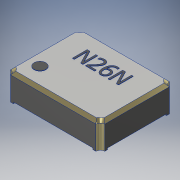
# Autodesk Inventor part: Crystal_TXO-3225
Saved by Autodesk Inventor 2018 (Build 220112000, 112)
## iProperties
Created: 2016-08-15
Part Number: Crystal_TXO-3225
Material: Aluminum 6061
Document SubType Name: Modeling
Designer: Bradley
Density: 2.7 g/cm^3
Appearance: Aluminum - Flat
Author: Bradley
Autodesk Inventor part; units mm, degrees
ref_plane "YZ Plane" through (0, 0, 0) normal (1, 0, 0) x (0, 1, 0)
ref_plane "XZ Plane" through (0, 0, 0) normal (0, 1, 0) x (-1, 0, 0)
ref_plane "XY Plane" through (0, 0, 0) normal (0, 0, 1) x (1, 0, 0)
sketch "Sketch1" plane through (0, 0, 0) normal (0, 1, 0) x (-1, 0, 0)
  line L0 (-1.6, 1.25) -> (1.6, 1.25)
  line L1 (1.6, 1.25) -> (1.6, -1.25)
  line L2 (1.6, -1.25) -> (-1.6, -1.25)
  line L3 (-1.6, -1.25) -> (-1.6, 1.25)
  line L4 (-1.6, 1.25) -> (1.6, -1.25) construction
  line L5 (1.6, 1.25) -> (-1.6, -1.25) construction
  arc A0 (1.6, -1.1) -> (1.45, -1.25) centre (1.6, -1.25) ccw
  arc A1 (-1.45, -1.25) -> (-1.6, -1.1) centre (-1.6, -1.25) ccw
  arc A2 (-1.6, 1.1) -> (-1.45, 1.25) centre (-1.6, 1.25) ccw
  arc A3 (1.45, 1.25) -> (1.6, 1.1) centre (1.6, 1.25) ccw
  point P0 (0, 0)
  dimension "d0" = 3.2
  dimension "d1" = 2.5
  dimension "d4" = 0.15
  constraints: 12 end point, 8 point on circle, 8 point on line, 4 centre point, 4 coincident, 3 equal radius, 2 midpoint, 2 parallel, 1 horizontal, 1 perpendicular
  measures "d0" distance of L1.end L2.end
  measures "d1" distance of L0.end L1.end
  measures "d4" radius of A0
extrude "Extrusion1" add sketch "Sketch1" along normal mid plane 0.85 contours L0 A3 L1 A0 L2 A1 L3 A2
chamfer "Chamfer1" distance 0.1 angle 45 8 edges at (0, 0.425, 1.25) (-1.4939, 0.425, 1.1439) (-1.6, 0.425, 0) (-1.4939, 0.425, -1.1439) (0, 0.425, -1.25) (1.4939, 0.425, -1.1439) (1.6, 0.425, 0) (1.4939, 0.425, 1.1439)
sketch "Sketch3" plane through (0, 0.425, 0) normal (0, 1, 0) x (1, 0, 0)
  line L0 (-1.3709, 1.15) -> (1.3709, 1.15) projected
  arc A0 (-1.5, 1.0209) -> (-1.3709, 1.15) centre (-1.6, 1.25) ccw projected
  line L1 (-1.5, -1.0209) -> (-1.5, 1.0209) projected
  arc A1 (-1.3709, -1.15) -> (-1.5, -1.0209) centre (-1.6, -1.25) ccw projected
  line L2 (1.3709, -1.15) -> (-1.3709, -1.15) projected
  arc A2 (1.5, -1.0209) -> (1.3709, -1.15) centre (1.6, -1.25) ccw projected
  line L3 (1.5, 1.0209) -> (1.5, -1.0209) projected
  arc A3 (1.3709, 1.15) -> (1.5, 1.0209) centre (1.6, 1.25) ccw projected
  line L4 (1.5, 1.0209) -> (1.5, -1.0209) construction
  line L5 (1.5, 0.1868) -> (-1.5, 0.1868) construction
  circle A4 centre (-1.1, -0.6) radius 0.2
  line L6 (-0.4259, 0.1868) -> (-0.5004, 0.1868)
  line L7 (-0.5004, 0.1868) -> (-0.7216, 0.6179)
  line L8 (-0.7216, 0.6179) -> (-0.7216, 0.1868)
  line L9 (-0.7216, 0.1868) -> (-0.7836, 0.1868)
  line L10 (-0.7836, 0.1868) -> (-0.7836, 0.6868)
  line L11 (-0.7836, 0.6868) -> (-0.6892, 0.6868)
  line L12 (-0.6892, 0.6868) -> (-0.4878, 0.2909)
  line L13 (-0.4878, 0.2909) -> (-0.4878, 0.6868)
  line L14 (-0.4878, 0.6868) -> (-0.4259, 0.6868)
  line L15 (-0.4259, 0.6868) -> (-0.4259, 0.1868)
  line L16 (-0.0304, 0.1868) -> (-0.3387, 0.1868)
  line L17 (-0.3387, 0.1868) -> (-0.3387, 0.2577)
  spline S0 degree 2 poles (-0.3387, 0.2577) (-0.3055, 0.2889) (-0.2464, 0.3468) (-0.218, 0.378) knots 0 0 0 1 2 2 2
  spline S1 degree 2 poles (-0.218, 0.378) (-0.1609, 0.4408) (-0.1191, 0.5162) (-0.1191, 0.5563) knots 0 0 0 1 2 2 2
  spline S2 degree 2 poles (-0.1191, 0.5563) (-0.1191, 0.5774) (-0.1321, 0.609) (-0.1438, 0.6191) knots 0 0 0 1 2 2 2
  spline S3 degree 2 poles (-0.1438, 0.6191) (-0.1556, 0.6292) (-0.1864, 0.6393) (-0.205, 0.6393) knots 0 0 0 1 2 2 2
  spline S4 degree 2 poles (-0.205, 0.6393) (-0.2229, 0.6393) (-0.2593, 0.6304) (-0.2759, 0.6235) knots 0 0 0 1 2 2 2
  spline S5 degree 2 poles (-0.2759, 0.6235) (-0.2901, 0.6179) (-0.3165, 0.6017) (-0.3246, 0.596) knots 0 0 0 1 2 2 2
  line L18 (-0.3246, 0.596) -> (-0.3282, 0.596)
  line L19 (-0.3282, 0.596) -> (-0.3282, 0.6673)
  spline S6 degree 2 poles (-0.3282, 0.6673) (-0.3075, 0.6774) (-0.2334, 0.6973) (-0.2002, 0.6973) knots 0 0 0 1 2 2 2
  spline S7 degree 2 poles (-0.2002, 0.6973) (-0.1301, 0.6973) (-0.0511, 0.6231) (-0.0511, 0.5599) knots 0 0 0 1 2 2 2
  spline S8 degree 2 poles (-0.0511, 0.5599) (-0.0511, 0.5304) (-0.0648, 0.4809) (-0.077, 0.4599) knots 0 0 0 1 2 2 2
  spline S9 degree 2 poles (-0.077, 0.4599) (-0.0891, 0.438) (-0.1244, 0.395) (-0.1438, 0.3744) knots 0 0 0 1 2 2 2
  spline S10 degree 2 poles (-0.1438, 0.3744) (-0.1754, 0.3399) (-0.2528, 0.2662) (-0.2759, 0.2447) knots 0 0 0 1 2 2 2
  line L20 (-0.2759, 0.2447) -> (-0.0304, 0.2447)
  line L21 (-0.0304, 0.2447) -> (-0.0304, 0.1868)
  spline S11 degree 2 poles (0.3525, 0.3488) (0.3525, 0.3103) (0.327, 0.2451) (0.3055, 0.2232) knots 0 0 0 1 2 2 2
  spline S12 degree 2 poles (0.3055, 0.2232) (0.2832, 0.2001) (0.2273, 0.1762) (0.1937, 0.1762) knots 0 0 0 1 2 2 2
  spline S13 degree 2 poles (0.1937, 0.1762) (0.16, 0.1762) (0.1045, 0.1989) (0.0835, 0.2216) knots 0 0 0 1 2 2 2
  spline S14 degree 2 poles (0.0835, 0.2216) (0.0575, 0.2488) (0.0284, 0.3399) (0.0284, 0.4064) knots 0 0 0 1 2 2 2
  spline S15 degree 2 poles (0.0284, 0.4064) (0.0284, 0.4716) (0.0551, 0.5765) (0.0831, 0.6154) knots 0 0 0 1 2 2 2
  spline S16 degree 2 poles (0.0831, 0.6154) (0.1102, 0.6535) (0.1961, 0.6961) (0.2524, 0.6961) knots 0 0 0 1 2 2 2
  spline S17 degree 2 poles (0.2524, 0.6961) (0.269, 0.6961) (0.2982, 0.6928) (0.3092, 0.6892) knots 0 0 0 1 2 2 2
  line L22 (0.3092, 0.6892) -> (0.3092, 0.6248)
  line L23 (0.3092, 0.6248) -> (0.3063, 0.6248)
  spline S18 degree 2 poles (0.3063, 0.6248) (0.297, 0.6296) (0.263, 0.6381) (0.2435, 0.6381) knots 0 0 0 1 2 2 2
  spline S19 degree 2 poles (0.2435, 0.6381) (0.1811, 0.6381) (0.1045, 0.5539) (0.0972, 0.4712) knots 0 0 0 1 2 2 2
  spline S20 degree 2 poles (0.0972, 0.4712) (0.1212, 0.4878) (0.1714, 0.506) (0.2014, 0.506) knots 0 0 0 1 2 2 2
  spline S21 degree 2 poles (0.2014, 0.506) (0.2306, 0.506) (0.2743, 0.4943) (0.2982, 0.4765) knots 0 0 0 1 2 2 2
  spline S22 degree 2 poles (0.2982, 0.4765) (0.3258, 0.4558) (0.3525, 0.3918) (0.3525, 0.3488) knots 0 0 0 1 2 2 2
  spline S23 degree 2 poles (0.2844, 0.346) (0.2844, 0.3768) (0.2682, 0.4185) (0.2504, 0.4331) knots 0 0 0 1 2 2 2
  spline S24 degree 2 poles (0.2504, 0.4331) (0.237, 0.4436) (0.2038, 0.4505) (0.1864, 0.4505) knots 0 0 0 1 2 2 2
  spline S25 degree 2 poles (0.1864, 0.4505) (0.1629, 0.4505) (0.1187, 0.4364) (0.0972, 0.423) knots 0 0 0 1 2 2 2
  spline S26 degree 2 poles (0.0972, 0.423) (0.0968, 0.4157) (0.096, 0.4019) (0.096, 0.3914) knots 0 0 0 1 2 2 2
  spline S27 degree 2 poles (0.096, 0.3914) (0.096, 0.3395) (0.1163, 0.2759) (0.1317, 0.2593) knots 0 0 0 1 2 2 2
  spline S28 degree 2 poles (0.1317, 0.2593) (0.1459, 0.2435) (0.1767, 0.2309) (0.1941, 0.2309) knots 0 0 0 1 2 2 2
  spline S29 degree 2 poles (0.1941, 0.2309) (0.2346, 0.2309) (0.2844, 0.2885) (0.2844, 0.346) knots 0 0 0 1 2 2 2
  line L24 (0.7836, 0.1868) -> (0.7091, 0.1868)
  line L25 (0.7091, 0.1868) -> (0.4878, 0.6179)
  line L26 (0.4878, 0.6179) -> (0.4878, 0.1868)
  line L27 (0.4878, 0.1868) -> (0.4259, 0.1868)
  line L28 (0.4259, 0.1868) -> (0.4259, 0.6868)
  line L29 (0.4259, 0.6868) -> (0.5203, 0.6868)
  line L30 (0.5203, 0.6868) -> (0.7216, 0.2909)
  line L31 (0.7216, 0.2909) -> (0.7216, 0.6868)
  line L32 (0.7216, 0.6868) -> (0.7836, 0.6868)
  line L33 (0.7836, 0.6868) -> (0.7836, 0.1868)
  point P0 (0, 0)
  dimension "d27" = 0.4
  dimension "d28" = 0.6
  dimension "d29" = 1.1
  constraints: 2 end point, 2 point on line, 1 centre point, 1 horizontal, 1 perpendicular
  measures "d27" diameter of A4
  measures "d28" vertical distance of point (0, 0) A4.centre
  measures "d29" horizontal distance of point (0, 0) A4.centre
extrude "Extrusion3" add sketch "Sketch3" along normal blind 0.01 contours A4 | L6 L7 L8 L9 L10 L11 L12 L13 L14 L15 | L16 L17 S0 S1 S2 S3 S4 S5 L18 L19 S6 S7 S8 S9 S10 L20 L21 | S11 S12 S13 S14 S15 S16 S17 L22 L23 S18 S19 S20 S21 S22 | L24 L25 L26 L27 L28 L29 L30 L31 L32 L33
sketch "Sketch4" plane through (0, -0.425, 0) normal (0, -1, 0) x (1, 0, 0)
  line L0 (-1.6, 1.1) -> (-1.6, -1.1) projected
  arc A0 (-1.45, -1.25) -> (-1.6, -1.1) centre (-1.6, -1.25) ccw projected
  line L1 (-1.45, -1.25) -> (1.45, -1.25) projected
  arc A1 (1.6, -1.1) -> (1.45, -1.25) centre (1.6, -1.25) ccw projected
  line L2 (1.6, -1.1) -> (1.6, 1.1) projected
  arc A2 (1.45, 1.25) -> (1.6, 1.1) centre (1.6, 1.25) ccw projected
  line L3 (1.45, 1.25) -> (-1.45, 1.25) projected
  arc A3 (-1.6, 1.1) -> (-1.45, 1.25) centre (-1.6, 1.25) ccw projected
  line L4 (1.35, 1.25) -> (1.35, 1.19)
  line L5 (1.35, 1.19) -> (0.94, 1.19)
  line L6 (0.94, 1.19) -> (0.94, 0.35)
  line L7 (0.94, 0.35) -> (1.54, 0.35)
  line L8 (1.54, 0.35) -> (1.54, 1)
  line L9 (1.54, 1) -> (1.6, 1)
  line L10 (-1.6, -1.1) -> (-1.6, 1.1) projected
  line L11 (-1.6, 1) -> (-1.54, 1)
  line L12 (-1.54, 1) -> (-1.54, 0.35)
  line L13 (-1.54, 0.35) -> (-0.94, 0.35)
  line L14 (-0.94, 0.35) -> (-0.94, 1.19)
  line L15 (-0.94, 1.19) -> (-1.35, 1.19)
  line L16 (-1.35, 1.19) -> (-1.35, 1.25)
  line L17 (1.45, -1.25) -> (-1.45, -1.25) projected
  line L18 (-1.35, -1.25) -> (-1.35, -1.19)
  line L19 (-1.35, -1.19) -> (-0.94, -1.19)
  line L20 (-0.94, -1.19) -> (-0.94, -0.35)
  line L21 (-0.94, -0.35) -> (-1.54, -0.35)
  line L22 (-1.54, -0.35) -> (-1.54, -1)
  line L23 (-1.54, -1) -> (-1.6, -1)
  line L24 (1.6, -1) -> (1.54, -1)
  line L25 (1.54, -1) -> (1.54, -0.35)
  line L26 (1.54, -0.35) -> (0.94, -0.35)
  line L27 (0.94, -0.35) -> (0.94, -1.19)
  line L28 (0.94, -1.19) -> (1.35, -1.19)
  line L29 (1.35, -1.19) -> (1.35, -1.25)
  point P0 (0, 0)
  dimension "d20" = 0.84
  dimension "d21" = 0.6
  dimension "d22" = 1.88
  dimension "d23" = 0.25
  dimension "d24" = 0.25
  constraints: 48 end point, 20 point on line, 15 perpendicular, 7 equal length, 6 collinear, 1 horizontal, 1 parallel, 1 vertical
  measures "d20" distance of L5.end L6.end
  measures "d21" distance of L6.end L7.end
  measures "d22" distance between parallel lines of L14 L6
  measures "d23" distance between parallel lines of L4 L2
  measures "d24" distance between parallel lines of L9 L3
extrude "Extrusion5" add sketch "Sketch4" along normal blind 0.05 contours A3 L3 L16 L15 L14 L13 L12 L11 L0 | L23 L22 L21 L20 L19 L18 L1 A0 L0 | L3 A2 L2 L9 L8 L7 L6 L5 L4 | L29 L28 L27 L26 L25 L24 L2 A1 L1
equation "\"d24\" = d23"
body "Solid1"
